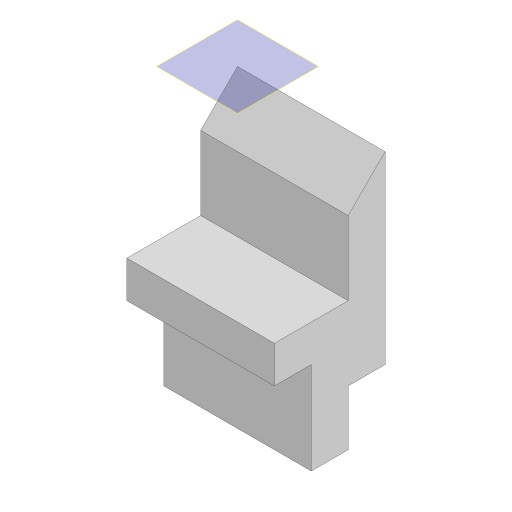
# Autodesk Inventor part: vistas_ortogonais
Saved by Autodesk Inventor 2024.3 (Build 283343000, 343)
## iProperties
Created: 2025-02-04
Part Number: vistas_ortogonais
Material: Generic
Document SubType Name: Modeling
Designer: Fernando.Molina
Density: 1 g/cm^3
Appearance: Default
Author: FMJ
Title: DESENHO TÉCNICO ASSISTIDO POR COMPUTADOR
Subject: UNIVESP
Autodesk Inventor part; units mm, degrees
ref_plane "YZ Plane" through (0, 0, 0) normal (1, 0, 0) x (0, 1, 0)
ref_plane "XZ Plane" through (0, 0, 0) normal (0, 1, 0) x (-1, 0, 0)
ref_plane "XY Plane" through (0, 0, 0) normal (0, 0, 1) x (1, 0, 0)
sketch "Sketch1" plane through (0, 0, 0) normal (1, 0, 0) x (0, 1, 0)
  line L0 (-10, 0) -> (-10, 15)
  line L1 (-10, 15) -> (0, 15)
  line L2 (0, 15) -> (0, 65)
  line L3 (0, 65) -> (-10, 55)
  line L4 (-10, 55) -> (-10, 35)
  line L5 (-10, 35) -> (-30, 35)
  line L6 (-30, 35) -> (-30, 25)
  line L7 (-30, 25) -> (-20, 25)
  line L8 (-20, 25) -> (-20, 0)
  line L9 (-20, 0) -> (-10, 0)
  point P0 (0, 0)
  dimension "d0" = 65
  dimension "d1" = 15
  dimension "d2" = 10
  dimension "d3" = 10
  dimension "d4" = 10
  dimension "d5" = 25
  dimension "d6" = 10
  dimension "d7" = 20
  constraints: 20 end point, 7 perpendicular, 4 point on line, 1 vertical
  measures "d0" distance from line of L2.end L9
  measures "d1" distance between parallel lines of L1 L9
  measures "d2" distance between parallel lines of L0 L2
  measures "d3" distance between parallel lines of L8 L0
  measures "d4" distance between parallel lines of L6 L8
  measures "d5" distance between parallel lines of L7 L9
  measures "d6" distance between parallel lines of L5 L7
  measures "d7" distance from line of L3.end L5
extrude "Extrusion1" add sketch "Sketch1" along normal mid plane 40
ref_plane "Work Plane1" through (-20, 0, 65) normal (0, 0, -1) x (-1, 0, 0)
body "Solid1"
